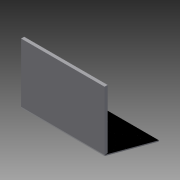
# Autodesk Inventor part: laptop
Saved by Autodesk Inventor 2017 (Build 210142000, 142)
## iProperties
Created: 2018-10-12
Part Number: laptop
Material: PC/ABS Plastic
Document SubType Name: Modeling
Designer: ari
Mass: 517.646 g
Surface Area: 3263.84 cm^2
Volume: 1448.88 cm^3
Density: 0.357273 g/cm^3
Appearance: Smooth - White
Author: ari
Autodesk Inventor part; units mm, degrees
ref_plane "YZ Plane" through (0, 0, 0) normal (1, 0, 0) x (0, 1, 0)
ref_plane "XZ Plane" through (0, 0, 0) normal (0, 1, 0) x (-1, 0, 0)
ref_plane "XY Plane" through (0, 0, 0) normal (0, 0, 1) x (1, 0, 0)
sketch "Sketch1" plane through (0, 0, 0) normal (1, 0, 0) x (0, 1, 0)
  line L0 (1.0353, 0) -> (210.6412, -56.1637)
  line L1 (210.6412, -56.1637) -> (209.6059, -60.0274)
  line L2 (209.6059, -60.0274) -> (0, -3.8637)
  line L3 (0, -3.8637) -> (1.0353, 0)
  line L4 (0, -72.0329) -> (0, 12.0055) construction
  line L5 (-42.1282, 0) -> (252.7694, 0) construction
  point P0 (0, 0)
  dimension "d0" = 217
  dimension "d1" = 4
  dimension "d2" = 75
  constraints: 8 end point, 2 parallel, 2 point on line, 1 perpendicular
  measures "d0" distance of L1.end L2.end
  measures "d1" distance of L2.end L0.start
  measures "d2" angle of L4 L2
extrude "Extrusion1" add sketch "Sketch1" along normal mid plane 323.5
sketch "Sketch2" plane through (0, 0, 0) normal (1, 0, 0) x (0, 1, 0)
  line L0 (0, 0) -> (12, 0)
  line L1 (12, 0) -> (12, 229)
  line L2 (12, 229) -> (0, 229)
  line L3 (0, 229) -> (0, 0)
  dimension "d5" = 229
  dimension "d6" = 12
  constraints: 8 end point, 2 parallel, 1 horizontal, 1 perpendicular
  measures "d5" distance of L2.end L0.start
  measures "d6" distance of L1.end L2.end
extrude "Extrusion2" add sketch "Sketch2" along normal mid plane 323.5
body "Solid1"
